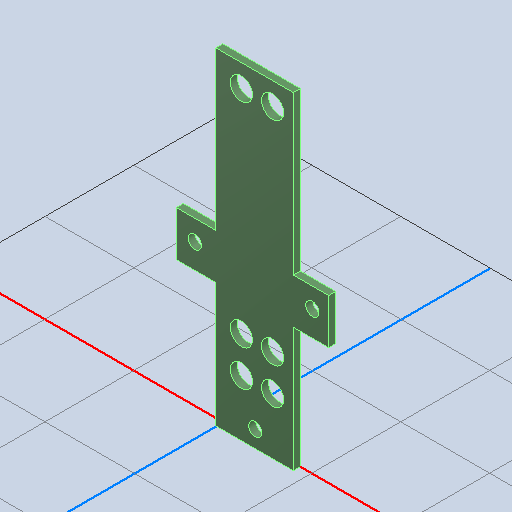
# Autodesk Inventor part: xt60_pcb.brdКонтур
Saved by Autodesk Inventor 2022 (Build 260153000, 153)
## iProperties
Created: 2023-01-24
Part Number: xt60_pcb.brdКонтур
Material: Типовые
Document SubType Name: Modeling
Designer: Иван Петров
Density: 1 g/cm^3
Appearance: Контур панели
Author: Иван Петров
Autodesk Inventor part; units mm, degrees
ref_plane "YZ Plane" through (0, 0, 0) normal (1, 0, 0) x (0, 1, 0)
ref_plane "XZ Plane" through (0, 0, 0) normal (0, 1, 0) x (-1, 0, 0)
ref_plane "XY Plane" through (0, 0, 0) normal (0, 0, 1) x (1, 0, 0)
sketch "Эскиз1" plane through (0, 0, 0) normal (0, 0, 1) x (1, 0, 0)
  line L0 (0, -8.89) -> (17.45, -8.89)
  line L1 (17.45, -8.89) -> (17.453, 19.05)
  line L2 (17.453, 19.05) -> (25.4, 19.05)
  line L3 (25.4, 19.05) -> (25.4, 29.21)
  line L4 (25.4, 29.21) -> (17.45, 29.21)
  line L5 (17.45, 29.21) -> (17.45, 64.76)
  line L6 (17.45, 64.76) -> (0, 64.76)
  line L7 (0, 64.76) -> (0, 29.21)
  line L8 (0, 29.21) -> (-8.89, 29.21)
  line L9 (-8.89, 29.21) -> (-8.89, 19.05)
  line L10 (-8.89, 19.05) -> (0, 19.05)
  line L11 (0, 19.05) -> (0, -8.89)
  circle A0 centre (5.77, 3.81) radius 2.5
  circle A1 centre (12.77, 3.81) radius 2.5
  circle A2 centre (5.77, 11.94) radius 2.5
  circle A3 centre (12.77, 11.94) radius 2.5
  circle A4 centre (5.77, 59.69) radius 2.5
  circle A5 centre (12.77, 59.69) radius 2.5
  circle A6 centre (8.89, -5.08) radius 1.5
  circle A7 centre (-4.699, 24.638) radius 1.5
  circle A8 centre (21.717, 24.765) radius 1.5
  constraints: 24 end point, 9 centre point
extrude "xt60_pcb.brdКонтур" add sketch "Эскиз1" along normal blind 1.6
